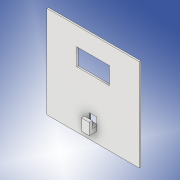
# Autodesk Inventor part: Top Cover
Saved by Autodesk Inventor 2017 SP1 (Build 210196100, 196)
## iProperties
Created: 2017-07-19
Part Number: Top Cover
Material: ABS Plastic
Document SubType Name: Modeling
Designer: zallen
Density: 1.06 g/cm^3
Appearance: CR White
Author: zallen
Autodesk Inventor part; units mm, degrees
ref_plane "YZ Plane" through (0, 0, 0) normal (1, 0, 0) x (0, 1, 0)
ref_plane "XZ Plane" through (0, 0, 0) normal (0, 1, 0) x (-1, 0, 0)
ref_plane "XY Plane" through (0, 0, 0) normal (0, 0, 1) x (1, 0, 0)
sketch "Sketch1" plane through (0, 0, 0) normal (0, 0, 1) x (1, 0, 0)
  line L0 (0, 0) -> (600, 0)
  line L1 (600, 0) -> (600, 600)
  line L2 (600, 600) -> (0, 600)
  line L3 (0, 600) -> (0, 0)
  dimension "d0" = 600
  dimension "d1" = 600
  constraints: 8 end point, 2 parallel, 1 horizontal, 1 perpendicular
  measures "d0" distance of L2.end L1.end
  measures "d1" distance of L1.end L0.end
extrude "Extrusion1" add sketch "Sketch1" along normal blind 10
sketch "Sketch2" plane through (0, 0, 10) normal (0, 0, 1) x (1, 0, 0)
  line L0 (193.5, 368) -> (406.5, 368)
  line L1 (406.5, 368) -> (406.5, 481)
  line L2 (406.5, 481) -> (193.5, 481)
  line L3 (193.5, 481) -> (193.5, 368)
  line L4 (0, 600) -> (0, 0) projected
  line L5 (600, 600) -> (0, 600) projected
  dimension "d4" = 213
  dimension "d5" = 113
  dimension "d6" = 193.5
  dimension "d7" = 119
  constraints: 8 end point, 2 parallel, 1 horizontal, 1 perpendicular
  measures "d4" distance of L2.end L1.end
  measures "d5" distance of L1.end L0.end
  measures "d6" distance between parallel lines of L4 L3
  measures "d7" distance from line of L5 L2.end
extrude "Extrusion2" cut sketch "Sketch2" against normal through all
sketch "Sketch3" plane through (0, 0, 10) normal (0, 0, 1) x (1, 0, 0)
  circle A0 centre (144.1129, 397.844) radius 80 construction
  circle A1 centre (455.8871, 397.844) radius 80 construction
  line L0 (220, 501) -> (380, 501)
  line L1 (380, 501) -> (338.589, 346.4519) construction
  line L2 (220, 501) -> (261.411, 346.4519) construction
  line L3 (261.411, 346.4519) -> (338.589, 346.4519)
  line L4 (123.4074, 475.1181) -> (220, 501)
  line L5 (261.411, 346.4519) -> (164.8185, 320.57)
  arc A2 (123.4074, 475.1181) -> (164.8185, 320.57) centre (144.1129, 397.844) ccw
  line L6 (380, 501) -> (476.5926, 475.1181)
  line L7 (338.589, 346.4519) -> (435.1815, 320.57)
  arc A3 (435.1815, 320.57) -> (476.5926, 475.1181) centre (455.8871, 397.844) ccw
  line L8 (193.5, 481) -> (406.5, 481) projected
  point P0 (0, 0)
  point P1 (424.4703, 324.271)
  point P2 (300, 481)
  point P3 (300, 501)
  dimension "d10" = 160
  dimension "d11" = 160
  dimension "d12" = 160
  dimension "d13" = 160
  dimension "d14" = 160
  dimension "d15" = 75
  dimension "d16" = 75
  dimension "d17" = 100
  dimension "d18" = 100
  dimension "d19" = 20
  constraints: 16 end point, 9 point on circle, 6 tangent, 4 centre point, 2 midpoint, 2 parallel, 1 concentric, 1 horizontal, 1 vertical alignment
  measures "d10" diameter of A0
  measures "d11" diameter of A1
  measures "d12" distance of L0.start L0.end
  measures "d13" distance of L0.end L1.end
  measures "d14" distance of L0.start L2.end
  measures "d15" angle of L0 L2
  measures "d16" angle of L0 L1
  measures "d17" distance of L4.start L0.start
  measures "d18" distance of L0.end L6.end
  measures "d19" distance between parallel lines of L0 L8
extrude "Extrusion3" [suppressed]
sketch "Sketch4" plane through (0, 0, 10) normal (0, 0, 1) x (1, 0, 0)
  line L0 (275, 150) -> (325, 150)
  line L1 (325, 150) -> (325, 100)
  line L2 (325, 100) -> (275, 100)
  line L3 (275, 100) -> (275, 150)
  line L4 (0, 0) -> (600, 0) projected
  point P0 (300, 100)
  point P1 (300, 0)
  dimension "d22" = 50
  dimension "d23" = 50
  dimension "d24" = 100
  constraints: 8 end point, 2 midpoint, 2 parallel, 1 horizontal, 1 perpendicular, 1 vertical alignment
  measures "d22" distance of L1.end L2.end
  measures "d23" distance of L0.end L1.end
  measures "d24" distance between parallel lines of L4 L2
extrude "Extrusion4" cut sketch "Sketch4" against normal through all
sketch "Sketch5" plane through (0, 0, 10) normal (0, 0, 1) x (1, 0, 0)
  line L0 (275, 100) -> (325, 100)
  line L1 (325, 100) -> (325, 70)
  line L2 (325, 70) -> (275, 70)
  line L3 (275, 70) -> (275, 100)
  point P0 (0, 0)
  dimension "d27" = 50
  dimension "d28" = 30
  constraints: 8 end point, 2 parallel, 1 coincident, 1 horizontal, 1 perpendicular
  measures "d27" distance of L1.end L2.end
  measures "d28" distance of L0.end L1.end
extrude "Extrusion5" add sketch "Sketch5" along normal blind 30
sketch "Sketch6" plane through (0, 0, 40) normal (0, 0, 1) x (1, 0, 0)
  line L0 (275, 70) -> (275, 100) projected
  line L1 (275, 70) -> (325, 70)
  line L2 (325, 70) -> (325, 145)
  line L3 (325, 145) -> (275, 145)
  line L4 (275, 145) -> (275, 70)
  point P0 (0, 0)
  dimension "d31" = 50
  dimension "d32" = 75
  constraints: 8 end point, 2 parallel, 1 horizontal, 1 perpendicular
  measures "d31" distance of L3.end L2.end
  measures "d32" distance of L2.end L1.end
extrude "Extrusion6" add sketch "Sketch6" along normal blind 20
body "Solid1"
